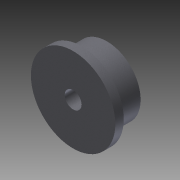
# Autodesk Inventor part: 2.5ingear proxy
Saved by Autodesk Inventor 2011 SP1 (Build 150282100, 282)
## iProperties
Created: 2012-01-20
Part Number: 2.5ingear proxy
Document SubType Name: Modeling
Designer: Christopher
Density: 1 g/cm^3
Author: Christopher
Autodesk Inventor part; units mm, degrees
ref_plane "YZ Plane" through (0, 0, 0) normal (1, 0, 0) x (0, 1, 0)
ref_plane "XZ Plane" through (0, 0, 0) normal (0, 1, 0) x (-1, 0, 0)
ref_plane "XY Plane" through (0, 0, 0) normal (0, 0, 1) x (1, 0, 0)
sketch "Sketch1" plane through (0, 0, 0) normal (0, 0, 1) x (1, 0, 0)
  circle A0 centre (0, 0) radius 31.75
  circle A1 centre (0, 0) radius 25.4
  circle A2 centre (0, 0) radius 6.35
  dimension "d0" = 63.5
  dimension "d1" = 50.8
  dimension "d2" = 12.7
  constraints: 3 centre point, 3 coincident
  measures "d0" diameter of A0
  measures "d1" diameter of A1
  measures "d2" diameter of A2
extrude "Extrusion1" add sketch "Sketch1" along normal blind 6.35 contours A0
extrude "Extrusion2" add sketch "Sketch1" along normal blind 6.35 contours A1
extrude "Extrusion3" add sketch "Sketch1" against normal blind 19.05 contours A1
body "Solid1"
